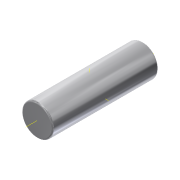
# Autodesk Inventor part: empty
Saved by Autodesk Inventor 2014 (Build 180170000, 170)
## iProperties
Created: 2015-04-13
Part Number: empty
Material: Generic
Document SubType Name: Modeling
Designer: Martin
Density: 1 g/cm^3
Appearance: Default
Author: Martin
Autodesk Inventor part; units mm, degrees
ref_plane "YZ Plane" through (0, 0, 0) normal (1, 0, 0) x (0, 1, 0)
ref_plane "XZ Plane" through (0, 0, 0) normal (0, 1, 0) x (-1, 0, 0)
ref_plane "XY Plane" through (0, 0, 0) normal (0, 0, 1) x (1, 0, 0)
sketch "Sketch1" plane through (0, 0, 0) normal (0, 1, 0) x (-1, 0, 0)
  circle A0 centre (0, 0) radius 0.78
  dimension "d0" = 1.56
  constraints: 1 centre point, 1 coincident
  measures "d0" diameter of A0
extrude "Extrusion1" add sketch "Sketch1" along normal mid plane 5.3
fillet "Fillet1" radius 0.08 2 edges at (0.78, -2.65, 0) (0.78, 2.65, 0)
body "Solid1"
